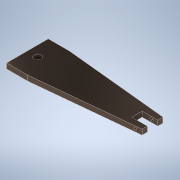
# Autodesk Inventor part: 4. 托板
Saved by Autodesk Inventor 2022 (Build 260153000, 153)
## iProperties
Created: 2023-05-12
Part Number: 4. 托板
Material: 一般
Document SubType Name: Modeling
Designer: USER
Density: 1 g/cm^3
Appearance: 砲銅 - 古董色拋光
Author: USER
Autodesk Inventor part; units mm, degrees
ref_plane "YZ Plane" through (0, 0, 0) normal (1, 0, 0) x (0, 1, 0)
ref_plane "XZ Plane" through (0, 0, 0) normal (0, 1, 0) x (-1, 0, 0)
ref_plane "XY Plane" through (0, 0, 0) normal (0, 0, 1) x (1, 0, 0)
sketch "草圖1" plane through (0, 0, 0) normal (0, 1, 0) x (-1, 0, 0)
  circle A0 centre (0, 0) radius 3.5
  line L0 (10, 20) -> (-10, 20)
  line L1 (-10, 20) -> (-10, -20)
  line L2 (-10, -20) -> (10, -20)
  line L3 (10, -20) -> (10, 20)
  line L4 (10, 20) -> (-10, -20) construction
  line L5 (-10, 20) -> (10, -20) construction
  line L6 (-95, 0) -> (-95, 5)
  line L7 (-95, 5) -> (-95, -5)
  line L8 (-95, -5) -> (-110, -5)
  line L9 (-110, -5) -> (-110, -10)
  line L10 (-110, -10) -> (-10, -20)
  line L11 (-95, -5) -> (-95, 5)
  line L12 (-95, 5) -> (-110, 5)
  line L13 (-110, 5) -> (-110, 10)
  line L14 (-110, 10) -> (-10, 20)
  dimension "d0" = 7
  dimension "d1" = 20
  dimension "d2" = 40
  dimension "d8" = 20
  dimension "d9" = 10
  dimension "d10" = 120
  dimension "d11" = 15
  constraints: 30 end point, 2 midpoint, 2 parallel, 2 perpendicular, 2 vertical, 1 centre point, 1 coincident, 1 horizontal, 1 point on line
  measures "d0" diameter of A0
  measures "d1" distance of L2.end L1.end
  measures "d2" distance of L1.end L0.end
  measures "d8" distance of L9.end L14.start
  measures "d9" distance of L11.start L6.end
  measures "d10" horizontal distance of L14.start L0.start
  measures "d11" distance of L8.end L7.end
extrude "擠出1" add sketch "草圖1" along normal blind 5
sketch "草圖2" plane through (-10, 0, 20) normal (0, 0, 1) x (1, 0, 0)
  line L0 (20, 0) -> (120, 0) projected
  line L1 (120, 0) -> (114, 0)
  line L2 (114, 0) -> (114, 2.5)
  circle A0 centre (114, 2.5) radius 1.5
  point P0 (10, 0)
  dimension "d14" = 6
  dimension "d15" = 2.5
  dimension "d16" = 3
  constraints: 4 end point, 1 centre point, 1 coincident, 1 perpendicular, 1 point on line
  measures "d14" distance of L0.end L1.end
  measures "d15" distance of L1.end L2.end
  measures "d16" diameter of A0
extrude "擠出2" cut sketch "草圖2" against normal through all
